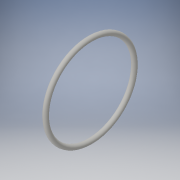
# Autodesk Inventor part: O-ring for LED Acrylic
Saved by Autodesk Inventor 2016 (Build 200138000, 138)
## iProperties
Created: 2017-09-28
Part Number: O-ring for LED Acrylic
Material: Generic
Document SubType Name: Modeling
Designer: Student
Density: 1 g/cm^3
Appearance: Default
Author: Student
Autodesk Inventor part; units mm, degrees
ref_plane "YZ Plane" through (0, 0, 0) normal (1, 0, 0) x (0, 1, 0)
ref_plane "XZ Plane" through (0, 0, 0) normal (0, 1, 0) x (-1, 0, 0)
ref_plane "XY Plane" through (0, 0, 0) normal (0, 0, 1) x (1, 0, 0)
sketch "Sketch1" plane through (0, 0, 0) normal (0, 1, 0) x (-1, 0, 0)
  line L0 (10.5791, 0) -> (-7.258, 0) construction
  circle A0 centre (3.6383, -24.8285) radius 1.3335
  point P0 (0, 0)
  dimension "d0" = 2.667
  dimension "d1" = 23.495
  constraints: 2 end point, 1 centre point, 1 horizontal
  measures "d0" diameter of A0
  measures "d1" distance edge to line of A0 L0
revolve "Revolution1" add sketch "Sketch1" angle 360 about axis through (-10.5791, 0, 0) along (1, 0, 0)
body "Solid1"
